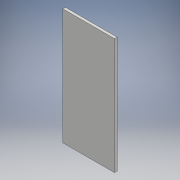
# Autodesk Inventor part: laterales
Saved by Autodesk Inventor 2018 (Build 220112000, 112)
## iProperties
Created: 2019-02-27
Part Number: laterales
Material: Genérico
Document SubType Name: Modeling
Designer: USUARIO WINDOWS
Density: 1 g/cm^3
Appearance: Valor por defecto
Author: USUARIO WINDOWS
Autodesk Inventor part; units mm, degrees
ref_plane "YZ Plane" through (0, 0, 0) normal (1, 0, 0) x (0, 1, 0)
ref_plane "XZ Plane" through (0, 0, 0) normal (0, 1, 0) x (-1, 0, 0)
ref_plane "XY Plane" through (0, 0, 0) normal (0, 0, 1) x (1, 0, 0)
sketch "Boceto1" plane through (0, 0, 0) normal (0, 1, 0) x (-1, 0, 0)
  line L0 (0, 0) -> (-64, 0)
  line L1 (-64, 0) -> (-64, -140)
  line L2 (-64, -140) -> (0, -140)
  line L3 (0, -140) -> (0, 0)
  dimension "d0" = 64
  dimension "d1" = 140
  constraints: 8 end point, 2 parallel, 1 horizontal, 1 perpendicular
  measures "d0" distance of L2.end L1.end
  measures "d1" distance of L1.end L0.end
extrude "Extrusión1" add sketch "Boceto1" along normal blind 3
sketch "Boceto2" plane through (64, 0, 0) normal (1, 0, 0) x (0, 0, -1)
  line L0 (0, 0) -> (140, 0) projected
  line L1 (140, 0) -> (140, 3) projected
  line L2 (0, 3) -> (140, 3) projected
  line L3 (0, 0) -> (0, 3) projected
extrude "Extrusión2" cut sketch "Boceto2" against normal blind 4
sketch "Boceto3" plane through (0, 0, 0) normal (0, 0, 1) x (1, 0, 0)
  line L0 (60, 0) -> (60, 3) projected
  line L1 (0, 3) -> (60, 3) projected
  line L2 (0, 0) -> (0, 3) projected
  line L3 (0, 0) -> (60, 0) projected
extrude "Extrusión3" cut sketch "Boceto3" along normal blind 5
sketch "Boceto4" plane through (0, 0, 0) normal (0, 0, 1) x (1, 0, 0)
  line L0 (60, 0) -> (60, 3) projected
  line L1 (0, 3) -> (60, 3) projected
  line L2 (0, 0) -> (0, 3) projected
  line L3 (0, 0) -> (60, 0) projected
extrude "Extrusión4" cut sketch "Boceto4" against normal blind 5
